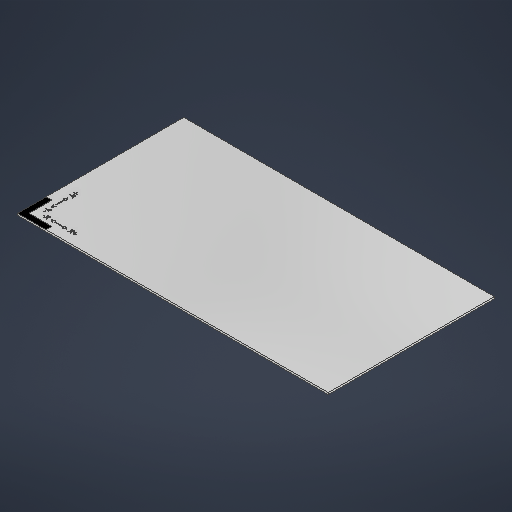
# Autodesk Inventor part: Base Plate
Saved by Autodesk Inventor 2025.1 (Build 291241000, 241)
## iProperties
Created: 2024-10-26
Part Number: Base Plate
Material: Generic
Document SubType Name: Modeling
Designer: jerem
Density: 1 g/cm^3
Appearance: Default
Author: jerem
Autodesk Inventor part; units mm, degrees
ref_plane "YZ Plane" through (0, 0, 0) normal (1, 0, 0) x (0, 1, 0)
ref_plane "XZ Plane" through (0, 0, 0) normal (0, 1, 0) x (-1, 0, 0)
ref_plane "XY Plane" through (0, 0, 0) normal (0, 0, 1) x (1, 0, 0)
sketch "Sketch1" plane through (0, 0, 0) normal (0, 1, 0) x (-1, 0, 0)
  line L0 (-546.1, -292.1) -> (546.1, -292.1)
  line L1 (546.1, -292.1) -> (546.1, 292.1)
  line L2 (546.1, 292.1) -> (-546.1, 292.1)
  line L3 (-546.1, 292.1) -> (-546.1, -292.1)
  line L4 (-546.1, -292.1) -> (546.1, 292.1) construction
  line L5 (546.1, -292.1) -> (-546.1, 292.1) construction
  point P0 (0, 0)
  dimension "d0" = 1092.2
  dimension "d1" = 584.2
  constraints: 12 end point, 2 midpoint, 2 parallel, 1 horizontal, 1 perpendicular
  measures "d0" distance of L2.end L1.end
  measures "d1" distance of L1.end L0.end
extrude "Extrusion1" add sketch "Sketch1" along normal blind 6.5
sketch "Sketch2" plane through (0, 6.5, 0) normal (0, 1, 0) x (1, 0, 0)
  line L0 (-546.1, 292.1) -> (-546.1, -292.1) projected
  line L1 (-546.1, -192.1) -> (-526.1, -192.1)
  line L2 (-526.1, -192.1) -> (-526.1, -292.1)
  line L3 (-526.1, -292.1) -> (-446.1, -292.1)
  line L4 (-446.1, -292.1) -> (-446.1, -272.1)
  line L5 (-446.1, -272.1) -> (-526.1, -272.1)
  line L6 (-526.1, -292.1) -> (-546.1, -292.1)
  line L7 (-546.1, -292.1) -> (-546.1, -192.1)
  line L8 (-496.1, -242.1) -> (-376.1, -242.1) construction
  line L9 (-376.1, -242.1) -> (-376.1, -262.1) construction
  line L10 (-376.1, -262.1) -> (-496.1, -262.1) construction
  line L11 (-496.1, -262.1) -> (-496.1, -242.1) construction
  line L12 (-496.1, -122.1) -> (-496.1, -242.1) construction
  line L13 (-496.1, -242.1) -> (-516.1, -242.1) construction
  line L14 (-516.1, -242.1) -> (-516.1, -122.1) construction
  line L15 (-516.1, -122.1) -> (-496.1, -122.1) construction
  line L16 (-505.3382, -135.5319) -> (-505.3382, -130.4509)
  line L17 (-505.3382, -130.4509) -> (-510.4193, -130.4509)
  line L18 (-510.4193, -130.4509) -> (-510.4193, -128.7734)
  line L19 (-510.4193, -128.7734) -> (-505.3382, -128.7734)
  line L20 (-505.3382, -128.7734) -> (-505.3382, -123.6924)
  line L21 (-505.3382, -123.6924) -> (-503.7216, -123.6924)
  line L22 (-503.7216, -123.6924) -> (-503.7216, -128.7734)
  line L23 (-503.7216, -128.7734) -> (-498.6405, -128.7734)
  line L24 (-498.6405, -128.7734) -> (-498.6405, -130.4509)
  line L25 (-498.6405, -130.4509) -> (-503.7216, -130.4509)
  line L26 (-503.7216, -130.4509) -> (-503.7216, -135.5319)
  line L27 (-503.7216, -135.5319) -> (-505.3382, -135.5319)
  line L28 (-496.1, -149.134) -> (-504.463, -144.0652)
  line L29 (-504.463, -144.0652) -> (-511.1, -144.0652)
  line L30 (-511.1, -144.0652) -> (-511.1, -142.0716)
  line L31 (-511.1, -142.0716) -> (-504.6697, -142.0716)
  line L32 (-504.6697, -142.0716) -> (-496.1, -137.0028)
  line L33 (-496.1, -137.0028) -> (-496.1, -139.2151)
  line L34 (-496.1, -139.2151) -> (-502.7005, -143.0806)
  line L35 (-502.7005, -143.0806) -> (-496.1, -147.019)
  line L36 (-496.1, -147.019) -> (-496.1, -149.134)
  line L37 (-510.3099, -168.2912) -> (-505.1438, -157.4728)
  line L38 (-505.1438, -157.4728) -> (-503.9404, -157.4728)
  line L39 (-503.9404, -157.4728) -> (-498.7742, -168.2912)
  line L40 (-498.7742, -168.2912) -> (-500.5611, -168.2912)
  line L41 (-500.5611, -168.2912) -> (-504.536, -159.9039)
  line L42 (-504.536, -159.9039) -> (-508.523, -168.2912)
  line L43 (-508.523, -168.2912) -> (-510.3099, -168.2912)
  line L44 (-505.4476, -177.0433) -> (-505.4476, -171.3666)
  line L45 (-505.4476, -171.3666) -> (-503.6243, -171.3666)
  line L46 (-503.6243, -171.3666) -> (-503.6243, -177.0433)
  line L47 (-503.6243, -177.0433) -> (-505.4476, -177.0433)
  line L48 (-505.4476, -184.5311) -> (-505.4476, -178.8545)
  line L49 (-505.4476, -178.8545) -> (-503.6243, -178.8545)
  line L50 (-503.6243, -178.8545) -> (-503.6243, -184.5311)
  line L51 (-503.6243, -184.5311) -> (-505.4476, -184.5311)
  line L52 (-505.4476, -192.019) -> (-505.4476, -186.3423)
  line L53 (-505.4476, -186.3423) -> (-503.6243, -186.3423)
  line L54 (-503.6243, -186.3423) -> (-503.6243, -192.019)
  line L55 (-503.6243, -192.019) -> (-505.4476, -192.019)
  line L56 (-505.4476, -199.5068) -> (-505.4476, -193.8301)
  line L57 (-505.4476, -193.8301) -> (-503.6243, -193.8301)
  line L58 (-503.6243, -193.8301) -> (-503.6243, -199.5068)
  line L59 (-503.6243, -199.5068) -> (-505.4476, -199.5068)
  line L60 (-505.1438, -213.3885) -> (-510.3099, -202.57)
  line L61 (-510.3099, -202.57) -> (-508.523, -202.57)
  line L62 (-508.523, -202.57) -> (-504.536, -210.9574)
  line L63 (-504.536, -210.9574) -> (-500.5611, -202.57)
  line L64 (-500.5611, -202.57) -> (-498.7742, -202.57)
  line L65 (-498.7742, -202.57) -> (-503.9404, -213.3885)
  line L66 (-503.9404, -213.3885) -> (-505.1438, -213.3885)
  line L67 (-496.1, -233.8828) -> (-504.463, -228.8139)
  line L68 (-504.463, -228.8139) -> (-511.1, -228.8139)
  line L69 (-511.1, -228.8139) -> (-511.1, -226.8204)
  line L70 (-511.1, -226.8204) -> (-504.6697, -226.8204)
  line L71 (-504.6697, -226.8204) -> (-496.1, -221.7515)
  line L72 (-496.1, -221.7515) -> (-496.1, -223.9639)
  line L73 (-496.1, -223.9639) -> (-502.7005, -227.8293)
  line L74 (-502.7005, -227.8293) -> (-496.1, -231.7677)
  line L75 (-496.1, -231.7677) -> (-496.1, -233.8828)
  line L76 (-505.4476, -240.3374) -> (-505.4476, -234.6608)
  line L77 (-505.4476, -234.6608) -> (-503.6243, -234.6608)
  line L78 (-503.6243, -234.6608) -> (-503.6243, -240.3374)
  line L79 (-503.6243, -240.3374) -> (-505.4476, -240.3374)
  line L80 (-489.1652, -253.9476) -> (-494.8419, -253.9476)
  line L81 (-494.8419, -253.9476) -> (-494.8419, -252.1243)
  line L82 (-494.8419, -252.1243) -> (-489.1652, -252.1243)
  line L83 (-489.1652, -252.1243) -> (-489.1652, -253.9476)
  line L84 (-476.3776, -259.6) -> (-478.6628, -259.6)
  line L85 (-478.6628, -259.6) -> (-482.3095, -253.6194)
  line L86 (-482.3095, -253.6194) -> (-486.0291, -259.6)
  line L87 (-486.0291, -259.6) -> (-488.1806, -259.6)
  line L88 (-488.1806, -259.6) -> (-483.4035, -252.0878)
  line L89 (-483.4035, -252.0878) -> (-488.0348, -244.6)
  line L90 (-488.0348, -244.6) -> (-485.7495, -244.6)
  line L91 (-485.7495, -244.6) -> (-482.1758, -250.4712)
  line L92 (-482.1758, -250.4712) -> (-478.5291, -244.6)
  line L93 (-478.5291, -244.6) -> (-476.3776, -244.6)
  line L94 (-476.3776, -244.6) -> (-481.0696, -251.9906)
  line L95 (-481.0696, -251.9906) -> (-476.3776, -259.6)
  line L96 (-457.0015, -258.8099) -> (-467.82, -253.6438)
  line L97 (-467.82, -253.6438) -> (-467.82, -252.4404)
  line L98 (-467.82, -252.4404) -> (-457.0015, -247.2742)
  line L99 (-457.0015, -247.2742) -> (-457.0015, -249.0611)
  line L100 (-457.0015, -249.0611) -> (-465.3889, -253.036)
  line L101 (-465.3889, -253.036) -> (-457.0015, -257.023)
  line L102 (-457.0015, -257.023) -> (-457.0015, -258.8099)
  line L103 (-448.2495, -253.9476) -> (-453.9262, -253.9476)
  line L104 (-453.9262, -253.9476) -> (-453.9262, -252.1243)
  line L105 (-453.9262, -252.1243) -> (-448.2495, -252.1243)
  line L106 (-448.2495, -252.1243) -> (-448.2495, -253.9476)
  line L107 (-440.7617, -253.9476) -> (-446.4383, -253.9476)
  line L108 (-446.4383, -253.9476) -> (-446.4383, -252.1243)
  line L109 (-446.4383, -252.1243) -> (-440.7617, -252.1243)
  line L110 (-440.7617, -252.1243) -> (-440.7617, -253.9476)
  line L111 (-433.2738, -253.9476) -> (-438.9505, -253.9476)
  line L112 (-438.9505, -253.9476) -> (-438.9505, -252.1243)
  line L113 (-438.9505, -252.1243) -> (-433.2738, -252.1243)
  line L114 (-433.2738, -252.1243) -> (-433.2738, -253.9476)
  line L115 (-425.786, -253.9476) -> (-431.4626, -253.9476)
  line L116 (-431.4626, -253.9476) -> (-431.4626, -252.1243)
  line L117 (-431.4626, -252.1243) -> (-425.786, -252.1243)
  line L118 (-425.786, -252.1243) -> (-425.786, -253.9476)
  line L119 (-411.9043, -253.6438) -> (-422.7228, -258.8099)
  line L120 (-422.7228, -258.8099) -> (-422.7228, -257.023)
  line L121 (-422.7228, -257.023) -> (-414.3354, -253.036)
  line L122 (-414.3354, -253.036) -> (-422.7228, -249.0611)
  line L123 (-422.7228, -249.0611) -> (-422.7228, -247.2742)
  line L124 (-422.7228, -247.2742) -> (-411.9043, -252.4404)
  line L125 (-411.9043, -252.4404) -> (-411.9043, -253.6438)
  line L126 (-391.5437, -259.6) -> (-393.8289, -259.6)
  line L127 (-393.8289, -259.6) -> (-397.4756, -253.6194)
  line L128 (-397.4756, -253.6194) -> (-401.1952, -259.6)
  line L129 (-401.1952, -259.6) -> (-403.3468, -259.6)
  line L130 (-403.3468, -259.6) -> (-398.5696, -252.0878)
  line L131 (-398.5696, -252.0878) -> (-403.2009, -244.6)
  line L132 (-403.2009, -244.6) -> (-400.9156, -244.6)
  line L133 (-400.9156, -244.6) -> (-397.3419, -250.4712)
  line L134 (-397.3419, -250.4712) -> (-393.6952, -244.6)
  line L135 (-393.6952, -244.6) -> (-391.5437, -244.6)
  line L136 (-391.5437, -244.6) -> (-396.2357, -251.9906)
  line L137 (-396.2357, -251.9906) -> (-391.5437, -259.6)
  line L138 (-378.0267, -253.8382) -> (-383.1077, -253.8382)
  line L139 (-383.1077, -253.8382) -> (-383.1077, -258.9193)
  line L140 (-383.1077, -258.9193) -> (-384.7852, -258.9193)
  line L141 (-384.7852, -258.9193) -> (-384.7852, -253.8382)
  line L142 (-384.7852, -253.8382) -> (-389.8662, -253.8382)
  line L143 (-389.8662, -253.8382) -> (-389.8662, -252.2216)
  line L144 (-389.8662, -252.2216) -> (-384.7852, -252.2216)
  line L145 (-384.7852, -252.2216) -> (-384.7852, -247.1405)
  line L146 (-384.7852, -247.1405) -> (-383.1077, -247.1405)
  line L147 (-383.1077, -247.1405) -> (-383.1077, -252.2216)
  line L148 (-383.1077, -252.2216) -> (-378.0267, -252.2216)
  line L149 (-378.0267, -252.2216) -> (-378.0267, -253.8382)
  point P0 (0, 0)
  dimension "d4" = 20
  dimension "d5" = 20
  dimension "d6" = 100
  dimension "d7" = 100
  dimension "d8" = 120
  dimension "d9" = 120
  dimension "d10" = 20
  dimension "d11" = 20
  dimension "d12" = 10
  dimension "d13" = 10
  dimension "d14" = 30
  dimension "d15" = 30
  constraints: 14 end point, 5 perpendicular, 2 horizontal, 2 point on line, 4 other
  measures "d4" distance of L1.start L1.end
  measures "d5" distance of L3.end L4.end
  measures "d6" distance between parallel lines of L0 L4
  measures "d7" distance from line of L0.end L1
  measures "d8" distance of L13.end L14.end
  measures "d9" distance of L9.end L10.end
  measures "d10" distance of L10.end L8.start
  measures "d11" distance of L14.end L12.start
  measures "d12" distance between parallel lines of L2 L14
  measures "d13" distance between parallel lines of L5 L10
  measures "d14" distance between parallel lines of L2 L11
  measures "d15" distance between parallel lines of L5 L13
extrude "Extrusion2" cut sketch "Sketch2" against normal blind 0.5
equation "\"d5\" = d4"
body "Solid1"
